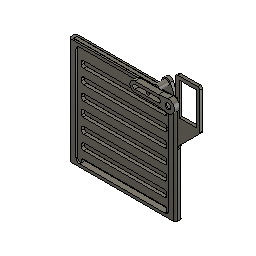
curtains (Autodesk Fusion 360 design; units mm, degrees)
Autodesk Fusion 360 part; units mm, degrees
note: some values were not read from the file. Chosen so that the rebuilt part matches the saved one: which bodies a step acts on; which face or edge a step refers to.
sketch "Sketch1" plane through (0, 0, 0) normal (0, 1, 0) x (1, 0, 0)
  line L0 (37.5, -2.5) -> (-37.5, -2.5)
  line L1 (-37.5, -2.5) -> (-37.5, 2.5)
  line L2 (-37.5, 2.5) -> (37.5, 2.5)
  line L3 (37.5, 2.5) -> (37.5, -2.5)
  line L4 (37.5, -2.5) -> (-37.5, 2.5) construction
  line L5 (-37.5, -2.5) -> (37.5, 2.5) construction
  dimension "d1" = 5
  dimension "d2" = 75
  constraint horizontal L0
  constraint perpendicular L0 L1
  constraint parallel L0 L2
  constraint parallel L1 L3
  constraint coincident L4 origin
  constraint coincident L5 origin
  measures "d1" distance of L0.end L1.end
  measures "d2" distance of L1.end L2.end
extrude "Extrude1" add sketch "Sketch1" along normal blind 75 makes body 1
sketch "Sketch2" plane through (0, 0, 2.5) normal (0, 0, 1) x (1, 0, 0)
  line L0 (-37.5, 0) -> (37.5, 0)
  line L1 (37.5, 0) -> (37.5, 75)
  line L2 (37.5, 75) -> (-37.5, 75)
  line L3 (-37.5, 75) -> (-37.5, 0)
  line L4 (-35.5, 2) -> (35.5, 2)
  line L5 (35.5, 2) -> (35.5, 73)
  line L6 (35.5, 73) -> (-35.5, 73)
  line L7 (-35.5, 73) -> (-35.5, 2)
  dimension "d5" = -2
extrude "Extrude2" cut sketch "Sketch2" against normal blind 3.8 contours L4 L5 L6 L7 bodies 1
sketch "Sketch3" plane through (0, 73, 0) normal (0, -1, 0) x (1, 0, 0)
  line L0 (35.5, 2.5) -> (-35.5, 2.5)
  line L1 (-35.5, 2.5) -> (-35.5, -1.3)
  line L2 (-35.5, -1.3) -> (35.5, -1.3)
  line L3 (35.5, -1.3) -> (35.5, 2.5)
  line L4 (35.5, 1.3) -> (-35.5, 1.3)
  dimension "d8" = 1.2
  constraint coincident L3 L4.start
  constraint coincident L1 L4.end
  constraint perpendicular L1 L4
  measures "d8" distance of L0 L4
extrude "Extrude3" cut sketch "Sketch3" against normal blind 5 contours L1 L2 L3 L4 bodies 1
sketch "Sketch4" plane through (0, 0, 2.5) normal (0, 0, 1) x (1, 0, 0)
  line L0 (35.5, 2) -> (-35.5, 2)
  line L1 (-35.5, 2) -> (-35.5, 73)
  line L2 (-35.5, 73) -> (35.5, 73)
  line L3 (35.5, 73) -> (35.5, 2)
  line L4 (-37.5, 0) -> (37.5, 0)
  line L5 (37.5, 0) -> (37.5, 75)
  line L6 (37.5, 75) -> (-37.5, 75)
  line L7 (-37.5, 75) -> (-37.5, 0)
  line L8 (-32.5, 73) -> (-32.5, 2)
  line L9 (32.5, 73) -> (32.5, 2)
  dimension "d11" = 3
  dimension "d12" = 3
  constraint coincident L2 L8.start
  constraint coincident L0 L8.end
  constraint perpendicular L0 L8
  constraint coincident L2 L9.start
  constraint coincident L0 L9.end
  constraint perpendicular L0 L9
  measures "d11" distance of L1 L8
  measures "d12" distance of L3 L9
extrude "Extrude4" add sketch "Sketch4" against normal blind 1.2 contours L0 L2 L3 L9 | L0 L1 L2 L8 bodies 1
sketch "Sketch5" plane through (0, 0, -1.3) normal (0, 0, 1) x (1, 0, 0)
  line L0 (-35.5, 75) -> (-35.5, 2)
  line L1 (-35.5, 2) -> (35.5, 2)
  line L2 (35.5, 2) -> (35.5, 75)
  line L3 (35.5, 75) -> (-35.5, 75)
  line L4 (-32.5, 73) -> (-32.5, 2)
  line L5 (32.5, 73) -> (32.5, 2)
  line L6 (32.5, 2) -> (-32.5, 2)
  line L7 (-32.5, 73) -> (32.5, 73)
  line L8 (0, 73) -> (0, 2) construction
  line L9 (30, 35) -> (-30, 35)
  line L10 (-30, 35) -> (-30, 40)
  line L11 (-30, 40) -> (30, 40)
  line L12 (30, 40) -> (30, 35)
  line L13 (30, 35) -> (-30, 40) construction
  line L14 (-30, 35) -> (30, 40) construction
  line L15 (30, 5) -> (-30, 5)
  line L16 (-30, 5) -> (-30, 10)
  line L17 (30, 10) -> (30, 5)
  line L18 (-30, 10) -> (30, 10)
  line L19 (30, 15) -> (-30, 15)
  line L20 (-30, 15) -> (-30, 20)
  line L21 (30, 20) -> (30, 15)
  line L22 (-30, 20) -> (30, 20)
  line L23 (30, 25) -> (-30, 25)
  line L24 (-30, 25) -> (-30, 30)
  line L25 (30, 30) -> (30, 25)
  line L26 (-30, 30) -> (30, 30)
  line L27 (30, 45) -> (-30, 45)
  line L28 (-30, 45) -> (-30, 50)
  line L29 (30, 50) -> (30, 45)
  line L30 (-30, 50) -> (30, 50)
  line L31 (30, 55) -> (-30, 55)
  line L32 (-30, 55) -> (-30, 60)
  line L33 (30, 60) -> (30, 55)
  line L34 (-30, 60) -> (30, 60)
  line L35 (30, 65) -> (-30, 65)
  line L36 (-30, 65) -> (-30, 70)
  line L37 (30, 70) -> (30, 65)
  line L38 (-30, 70) -> (30, 70)
  point P0 (0, 37.5)
  dimension "d15" = 60
  dimension "d16" = 5
  dimension "d19" = 0
  dimension "d20" = 10
  constraint midpoint L7 L8.start
  constraint midpoint L6 L8.end
  constraint horizontal L9
  constraint perpendicular L9 L10
  constraint parallel L9 L11
  constraint parallel L10 L12
  constraint coincident L13 P0
  constraint coincident L14 P0
  constraint midpoint L8 P0
  measures "d15" distance of L10.end L11.end
  measures "d16" distance of L9.end L10.end
extrude "Extrude5" cut sketch "Sketch5" against normal blind 5 contours L9 L10 L11 L12 | L15 L16 L17 L18 | L19 L20 L21 L22 | L23 L24 L25 L26 | L27 L28 L29 L30 | L31 L32 L33 L34 | L35 L36 L37 L38 bodies 1
fillet "Fillet1" radius 2.5 4 edges at (-32.5, 73, 1.9) (-32.5, 2, 1.9) (32.5, 73, 1.9) (32.5, 2, 1.9) on bodies 1
fillet "Fillet2" radius 1.5 4 edges at (-37.5, 37.5, 2.5) (-37.5, 37.5, -2.5) (37.5, 37.5, -2.5) (37.5, 37.5, 2.5) on bodies 1
fillet "Fillet3" radius 1.5 20 edges at (-30, 50, -1.9) (-30, 45, -1.9) (-30, 30, -1.9) (-30, 25, -1.9) (-30, 40, -1.9) (-30, 35, -1.9) (-30, 20, -1.9) (-30, 15, -1.9) (-30, 10, -1.9) (-30, 5, -1.9) (30, 50, -1.9) (30, 45, -1.9) (30, 30, -1.9) (30, 25, -1.9) (30, 40, -1.9) (30, 35, -1.9) (30, 20, -1.9) (30, 15, -1.9) (30, 10, -1.9) (30, 5, -1.9) on bodies 1
fillet "Fillet3" radius 1.5 8 edges at (-30, 55, -1.9) (-30, 60, -1.9) (-30, 65, -1.9) (-30, 70, -1.9) (30, 70, -1.9) (30, 65, -1.9) (30, 60, -1.9) (30, 55, -1.9) on bodies 1
sketch "Sketch6" plane through (0, 75, 0) normal (0, 1, 0) x (-1, 0, 0)
  arc A0 (-36, 2.5) -> (-37.5, 1) centre (-36, 1) ccw
  line L0 (-37.5, 1) -> (-37.5, -1)
  arc A1 (-37.5, -1) -> (-36, -2.5) centre (-36, -1) ccw
  line L1 (-36, -2.5) -> (36, -2.5)
  arc A2 (36, -2.5) -> (37.5, -1) centre (36, -1) ccw
  line L2 (37.5, -1) -> (37.5, 1)
  arc A3 (37.5, 1) -> (36, 2.5) centre (36, 1) ccw
  line L3 (36, 2.5) -> (-36, 2.5)
  line L4 (35.5, 1.3) -> (35.5, -1.3)
  line L5 (35.5, -1.3) -> (-35.5, -1.3)
  line L6 (-35.5, -1.3) -> (-35.5, 1.3)
  line L7 (-35.5, 1.3) -> (35.5, 1.3)
  line L8 (-35.3, 1.1) -> (35.3, 1.1)
  line L9 (35.3, 1.1) -> (35.3, -1.1)
  line L10 (35.3, -1.1) -> (-35.3, -1.1)
  line L11 (-35.3, -1.1) -> (-35.3, 1.1)
  dimension "d29" = 0.2
extrude "Extrude6" add sketch "Sketch6" against normal blind 73 separate body contours L8 L9 L10 L11 makes body 2
sketch "Sketch8" plane through (0, 0, 1.1) normal (0, 0, 1) x (1, 0, 0)
  line L0 (35.3, 75) -> (-35.3, 75)
  line L1 (-35.3, 75) -> (-35.3, 2)
  line L2 (-35.3, 2) -> (35.3, 2)
  line L3 (35.3, 2) -> (35.3, 75)
  line L4 (-28.5, 5) -> (28.5, 5)
  arc A0 (28.5, 5) -> (30, 6.5) centre (28.5, 6.5) ccw
  line L5 (30, 6.5) -> (30, 8.5)
  arc A1 (30, 8.5) -> (28.5, 10) centre (28.5, 8.5) ccw
  line L6 (28.5, 10) -> (-28.5, 10)
  arc A2 (-28.5, 10) -> (-30, 8.5) centre (-28.5, 8.5) ccw
  line L7 (-30, 8.5) -> (-30, 6.5)
  arc A3 (-30, 6.5) -> (-28.5, 5) centre (-28.5, 6.5) ccw
  line L8 (-28.5, 45) -> (28.5, 45)
  arc A4 (28.5, 45) -> (30, 46.5) centre (28.5, 46.5) ccw
  line L9 (30, 46.5) -> (30, 48.5)
  arc A5 (30, 48.5) -> (28.5, 50) centre (28.5, 48.5) ccw
  line L10 (28.5, 50) -> (-28.5, 50)
  arc A6 (-28.5, 50) -> (-30, 48.5) centre (-28.5, 48.5) ccw
  line L11 (-30, 48.5) -> (-30, 46.5)
  arc A7 (-30, 46.5) -> (-28.5, 45) centre (-28.5, 46.5) ccw
  line L12 (-28.5, 15) -> (28.5, 15)
  arc A8 (28.5, 15) -> (30, 16.5) centre (28.5, 16.5) ccw
  line L13 (30, 16.5) -> (30, 18.5)
  arc A9 (30, 18.5) -> (28.5, 20) centre (28.5, 18.5) ccw
  line L14 (28.5, 20) -> (-28.5, 20)
  arc A10 (-28.5, 20) -> (-30, 18.5) centre (-28.5, 18.5) ccw
  line L15 (-30, 18.5) -> (-30, 16.5)
  arc A11 (-30, 16.5) -> (-28.5, 15) centre (-28.5, 16.5) ccw
  line L16 (-28.5, 25) -> (28.5, 25)
  arc A12 (28.5, 25) -> (30, 26.5) centre (28.5, 26.5) ccw
  line L17 (30, 26.5) -> (30, 28.5)
  arc A13 (30, 28.5) -> (28.5, 30) centre (28.5, 28.5) ccw
  line L18 (28.5, 30) -> (-28.5, 30)
  arc A14 (-28.5, 30) -> (-30, 28.5) centre (-28.5, 28.5) ccw
  line L19 (-30, 28.5) -> (-30, 26.5)
  arc A15 (-30, 26.5) -> (-28.5, 25) centre (-28.5, 26.5) ccw
  line L20 (-30, 38.5) -> (-30, 36.5)
  arc A16 (-30, 36.5) -> (-28.5, 35) centre (-28.5, 36.5) ccw
  line L21 (-28.5, 35) -> (28.5, 35)
  arc A17 (28.5, 35) -> (30, 36.5) centre (28.5, 36.5) ccw
  line L22 (30, 36.5) -> (30, 38.5)
  arc A18 (30, 38.5) -> (28.5, 40) centre (28.5, 38.5) ccw
  line L23 (28.5, 40) -> (-28.5, 40)
  arc A19 (-28.5, 40) -> (-30, 38.5) centre (-28.5, 38.5) ccw
  line L24 (36, 75) -> (36, 0)
  line L25 (36, 0) -> (-36, 0)
  line L26 (-36, 0) -> (-36, 75)
  line L27 (-36, 75) -> (36, 75)
  line L28 (0, 45) -> (0, 30) construction
  line L29 (0, 25) -> (0, 40) construction
  line L30 (0, 35) -> (0, 20) construction
  line L31 (0, 15) -> (0, 10) construction
  line L32 (-30, 30.125) -> (30, 30.125)
  line L33 (30, 30.125) -> (30, 34.875)
  line L34 (30, 34.875) -> (-30, 34.875)
  line L35 (-30, 34.875) -> (-30, 30.125)
  line L36 (-30, 30.125) -> (30, 34.875) construction
  line L37 (30, 30.125) -> (-30, 34.875) construction
  line L38 (-30, 7.5) -> (30, 7.5) construction
  line L39 (30, 0.125) -> (30, 4.875)
  line L40 (30, 4.875) -> (-30, 4.875)
  line L41 (-30, 0.125) -> (30, 0.125)
  line L42 (-30, 4.875) -> (-30, 0.125)
  line L43 (30, 10.125) -> (30, 14.875)
  line L44 (30, 14.875) -> (-30, 14.875)
  line L45 (-30, 10.125) -> (30, 10.125)
  line L46 (-30, 14.875) -> (-30, 10.125)
  line L47 (30, 20.125) -> (30, 24.875)
  line L48 (30, 24.875) -> (-30, 24.875)
  line L49 (-30, 20.125) -> (30, 20.125)
  line L50 (-30, 24.875) -> (-30, 20.125)
  line L51 (30, 40.125) -> (30, 44.875)
  line L52 (30, 44.875) -> (-30, 44.875)
  line L53 (-30, 40.125) -> (30, 40.125)
  line L54 (-30, 44.875) -> (-30, 40.125)
  line L55 (30, 50.125) -> (30, 54.875)
  line L56 (30, 54.875) -> (-30, 54.875)
  line L57 (-30, 50.125) -> (30, 50.125)
  line L58 (-30, 54.875) -> (-30, 50.125)
  line L59 (30, 60.125) -> (30, 64.875)
  line L60 (30, 64.875) -> (-30, 64.875)
  line L61 (-30, 60.125) -> (30, 60.125)
  line L62 (-30, 64.875) -> (-30, 60.125)
  line L63 (30, 70.125) -> (30, 74.875)
  line L64 (30, 74.875) -> (-30, 74.875)
  line L65 (-30, 70.125) -> (30, 70.125)
  line L66 (-30, 74.875) -> (-30, 70.125)
  line L67 (-28.5, 65) -> (28.5, 65)
  line L68 (30, 66.5) -> (30, 68.5)
  line L69 (28.5, 70) -> (-28.5, 70)
  line L70 (-30, 68.5) -> (-30, 66.5)
  line L71 (-28.5, 55) -> (28.5, 55)
  line L72 (30, 56.5) -> (30, 58.5)
  line L73 (28.5, 60) -> (-28.5, 60)
  line L74 (-30, 58.5) -> (-30, 56.5)
  arc A20 (28.5, 65) -> (30, 66.5) centre (28.5, 66.5) ccw
  arc A21 (30, 68.5) -> (28.5, 70) centre (28.5, 68.5) ccw
  arc A22 (-28.5, 70) -> (-30, 68.5) centre (-28.5, 68.5) ccw
  arc A23 (-30, 66.5) -> (-28.5, 65) centre (-28.5, 66.5) ccw
  arc A24 (28.5, 55) -> (30, 56.5) centre (28.5, 56.5) ccw
  arc A25 (30, 58.5) -> (28.5, 60) centre (28.5, 58.5) ccw
  arc A26 (-28.5, 60) -> (-30, 58.5) centre (-28.5, 58.5) ccw
  arc A27 (-30, 56.5) -> (-28.5, 55) centre (-28.5, 56.5) ccw
  point P0 (0, 37.5)
  point P1 (0, 32.5)
  point P2 (0, 27.5)
  point P3 (0, 12.5)
  dimension "d36" = 4.75
  dimension "d39" = 60
  dimension "d54" = 0
  dimension "d55" = 10
  constraint midpoint L8 L28.start
  constraint midpoint L18 L28.end
  constraint midpoint L16 L29.start
  constraint midpoint L23 L29.end
  constraint midpoint L21 L30.start
  constraint midpoint L14 L30.end
  constraint midpoint L12 L31.start
  constraint midpoint L6 L31.end
  constraint midpoint L28 P0
  constraint horizontal L32
  constraint perpendicular L32 L33
  constraint parallel L32 L34
  constraint parallel L33 L35
  constraint coincident L36 P1
  constraint coincident L37 P1
  constraint midpoint L29 P1
  constraint midpoint L30 P2
  constraint midpoint L31 P3
  constraint midpoint L7 L38.start
  constraint midpoint L5 L38.end
  measures "d36" distance of L32.start L34.end
  measures "d39" distance of L33.end L34.end
extrude "Extrude8" cut sketch "Sketch8" against normal blind 2.2 contours L2 L39 L40 L42 | L32 L33 L34 L35 | L43 L44 L45 L46 | L47 L48 L49 L50 | L51 L52 L53 L54 | L55 L56 L57 L58 | L59 L60 L61 L62 bodies 2
fillet "Fillet4" radius 1 4 edges at (-30, 30.125, 0) (-30, 34.875, 0) (30, 34.875, 0) (30, 30.125, 0) on bodies 2
fillet "Fillet4" radius 1.5 22 edges at (-30, 24.875, 0) (-30, 20.125, 0) (-30, 14.875, 0) (-30, 10.125, 0) (-30, 4.875, 0) (30, 4.875, 0) (30, 10.125, 0) (30, 14.875, 0) (30, 20.125, 0) (30, 24.875, 0) (30, 44.875, 0) (30, 40.125, 0) (30, 54.875, 0) (30, 50.125, 0) (30, 64.875, 0) (30, 60.125, 0) (-30, 64.875, 0) (-30, 60.125, 0) (-30, 54.875, 0) (-30, 50.125, 0) (-30, 44.875, 0) (-30, 40.125, 0) on bodies 2
ref_plane "WorkPlane1" through (0, 37.5, 0) normal (0, 0, 1) x (1, 0, 0)
sketch "Sketch9" plane through (0, 25, 0) normal (0, 0, 1) x (1, 0, 0)
  line L0 (37.5, 50) -> (37.5, -25)
  line L1 (37.5, -25) -> (37.5, 50)
  line L2 (37.5, 50) -> (44.5, 50) construction
  line L3 (50.5, 38.5) -> (38.5, 38.5)
  line L4 (38.5, 38.5) -> (38.5, 61.5)
  line L5 (38.5, 61.5) -> (50.5, 61.5)
  line L6 (50.5, 61.5) -> (50.5, 38.5)
  line L7 (50.5, 38.5) -> (38.5, 61.5) construction
  line L8 (38.5, 38.5) -> (50.5, 61.5) construction
  line L9 (53, 36) -> (36, 36)
  line L10 (36, 36) -> (36, 64)
  line L11 (36, 64) -> (53, 64)
  line L12 (53, 64) -> (53, 36)
  point P0 (44.5, 50)
  dimension "d46" = 23
  dimension "d47" = 12
  dimension "d48" = 1
  dimension "d49" = -2.5
  constraint coincident L0.start L1.end
  constraint perpendicular L0 L2
  constraint horizontal L3
  constraint perpendicular L3 L4
  constraint parallel L3 L5
  constraint parallel L4 L6
  constraint coincident L7 P0
  constraint coincident L8 P0
  constraint coincident P0 L2.end
  measures "d46" distance of L3.start L5.end
  measures "d47" distance of L4.end L5.end
  measures "d48" distance of L1 L4
extrude "Extrude9" add sketch "Sketch9" along normal mid plane 2 bodies 1
chamfer "Chamfer1" distance 15.5 angle 45 1 edges at (37.5, 61, 0) on bodies 1
fillet "Fillet5" radius 5 1 edges at (37.5, 45.5031, 0) on bodies 1
fillet "Fillet6" radius 1.5 6 edges at (52.9984, 61, -1) (36, 89, 0) (52.9984, 61, 1) (52.9969, 61, 0) (53, 61, 0) (53, 89, 0) on bodies 1
sketch "Sketch10" plane through (0, 0, 1) normal (0, 0, 1) x (1, 0, 0)
  arc A0 (53, 87.5) -> (51.5, 89) centre (51.5, 87.5) ccw
  line L0 (51.5, 89) -> (37.5, 89)
  arc A1 (37.5, 89) -> (36, 87.5) centre (37.5, 87.5) ccw
  line L1 (36, 87.5) -> (36, 75)
  line L2 (36, 75) -> (37.5, 75)
  line L3 (37.5, 75) -> (37.5, 43.4289)
  arc A2 (38.9645, 46.9645) -> (37.5, 43.4289) centre (42.5, 43.4289) ccw
  line L4 (38.9645, 46.9645) -> (52.5607, 60.5607)
  line L5 (53, 61.6213) -> (53, 87.5)
  line L6 (38.5, 86.5) -> (50.5, 86.5)
  line L7 (50.5, 86.5) -> (50.5, 63.5)
  line L8 (50.5, 63.5) -> (38.5, 63.5)
  line L9 (38.5, 63.5) -> (38.5, 86.5)
  line L10 (44.5, 86.5) -> (44.5, 80.6)
  line L11 (44.5, 80.6) -> (29.5, 80.6) construction
  line L12 (35.3, 75) -> (-35.3, 75)
  line L13 (-35.3, 75) -> (35.3, 75)
  circle A3 centre (29.5, 80.6) radius 1
  circle A4 centre (29.5, 80.6) radius 3
  line L14 (35.3, 75) -> (32.2372, 81.8278)
  line L15 (29.5, 82.4332) -> (29.5, 78.4139) construction
  line L16 (23.7, 75) -> (26.7628, 81.8278)
  arc A5 (52.5607, 60.5607) -> (53, 61.6213) centre (51.5, 61.6213) ccw
  dimension "d65" = 15
  dimension "d66" = 5.9
  dimension "d67" = 2
  dimension "d68" = 2
  constraint midpoint L6 L10.start
  constraint perpendicular L6 L10
  constraint perpendicular L1 L11
  constraint coincident L11.end A3.centre
  constraint coincident L12.start L13.end
  constraint coincident A4 L14.end
  constraint tangent A4 L14
  constraint perpendicular L11 L15
  constraint symmetric L12.start L15 L16.start
  constraint symmetric L14.end L15 L16.end
  measures "d65" distance of L10.end L11.end
  measures "d66" distance of L6 L10.end
  measures "d67" diameter of A3
  measures "d68" distance of A3
extrude "Extrude10" add sketch "Sketch10" against normal blind 2.1 separate body contours L12 L13 A4 L14 L16 | A4 makes body 3
combine "Combine1" operation add target body 2 tool bodies 3
ref_plane "WorkPlane2" through (29.5, 79.3, 11) normal (0, 0, 1) x (1, 0, 0)
sketch "Sketch11" plane through (29.5, 79.3, 11) normal (0, 0, 1) x (1, 0, 0)
  circle A0 centre (0, 1.3) radius 1
  line L0 (9, 7.2) -> (21, 7.2)
  line L1 (9, -15.8) -> (9, 7.2)
  line L2 (21, -15.8) -> (9, -15.8)
  line L3 (21, 7.2) -> (21, -15.8)
  line L4 (15, 7.2) -> (15, 1.2) construction
  circle A1 centre (15, 1.2) radius 2.5
  line L5 (8.2797, 2.8) -> (-8.2797, 2.8)
  arc A2 (-8.2797, 2.8) -> (-8.2797, -0.2) centre (-8.2797, 1.3) ccw
  line L6 (-8.2797, -0.2) -> (8.2797, -0.2)
  arc A3 (8.2797, -0.2) -> (8.2797, 2.8) centre (8.2797, 1.3) ccw
  line L7 (8.2797, 1.3) -> (-8.2797, 1.3) construction
  line L8 (-8.2797, -2.2) -> (8.2797, -2.2)
  arc A4 (8.2797, -2.2) -> (8.2797, 4.8) centre (8.2797, 1.3) ccw
  line L9 (8.2797, 4.8) -> (-8.2797, 4.8)
  arc A5 (-8.2797, 4.8) -> (-8.2797, -2.2) centre (-8.2797, 1.3) ccw
  circle A6 centre (15, 1.2) radius 4.5
  line L10 (15, 5.7) -> (8.2797, 4.8)
  line L11 (15, -3.3) -> (8.2797, -2.2)
  point P0 (0, 1.3)
  dimension "d72" = 6
  dimension "d73" = 5
  dimension "d74" = 3
  dimension "d75" = 2
  dimension "d76" = 2
  constraint midpoint L0 L4.start
  constraint perpendicular L0 L4
  constraint coincident L4.end A1.centre
  constraint tangent L5 A2
  constraint tangent A2 L6
  constraint parallel L5 L6
  constraint tangent L6 A3
  constraint tangent L5 A3
  constraint horizontal L7
  constraint coincident P0 A0.centre
  constraint midpoint L7 P0
  constraint coincident A6 L10.start
  constraint coincident L4 L10.start
  constraint coincident A6 L11.start
  measures "d72" distance of L0 L4.end
  measures "d73" diameter of A1
  measures "d74" diameter of A2
extrude "Extrude11" add sketch "Sketch11" along normal blind 3 separate body contours L1 A4 A6 L10 | L1 A4 L10 | L1 A3 A4 A6 | L1 L5 A2 L6 A3 L8 A4 L9 A5 | A4 A6 L10 L11 | A4 A6 | L1 A4 L11 | L1 A4 A6 L11 makes body 4
sketch "Sketch12" plane through (0, 0, 14) normal (0, 0, 1) x (1, 0, 0)
  circle A0 centre (44.5, 80.5) radius 2.5
  arc A1 (37.7797, 79.1) -> (37.7797, 82.1) centre (37.7797, 80.6) ccw
  line L0 (37.7797, 79.1) -> (21.2203, 79.1)
  arc A2 (21.2203, 82.1) -> (21.2203, 79.1) centre (21.2203, 80.6) ccw
  line L1 (21.2203, 82.1) -> (37.7797, 82.1)
  line L2 (44.5, 85) -> (37.7797, 84.1)
  line L3 (37.7797, 84.1) -> (21.2203, 84.1)
  arc A3 (21.2203, 84.1) -> (21.2203, 77.1) centre (21.2203, 80.6) ccw
  line L4 (21.2203, 77.1) -> (37.7797, 77.1)
  line L5 (37.7797, 77.1) -> (44.5, 76)
  arc A4 (44.5, 76) -> (44.5, 85) centre (44.5, 80.5) ccw
  circle A5 centre (44.5, 80.5) radius 2
  dimension "d79" = 4
  constraint concentric A0 A5
  measures "d79" diameter of A5
extrude "Extrude12" add sketch "Sketch12" along normal blind 0.8 contours A0 | L2 L3 A3 L4 L5 A4 bodies 4
sketch "Sketch13" plane through (0, 0, 1) normal (0, 0, 1) x (1, 0, 0)
  circle A0 centre (29.5, 80.6) radius 1
  line L0 (35.3, 75) -> (32.2372, 81.8278)
  arc A1 (32.2372, 81.8278) -> (26.7628, 81.8278) centre (29.5, 80.6) ccw
  line L1 (26.7628, 81.8278) -> (23.7, 75)
  line L2 (23.7, 75) -> (35.3, 75)
  circle A2 centre (29.5, 80.6) radius 1
  circle A3 centre (29.5, 80.6) radius 2
  dimension "d82" = 2
  dimension "d83" = 4
  constraint concentric A0 A2
  constraint concentric A2 A3
  measures "d82" diameter of A2
  measures "d83" diameter of A3
extrude "Extrude13" add sketch "Sketch13" along normal blind 7 separate body contours A3 makes body 5
sketch "Sketch14" plane through (0, 0, 8) normal (0, 0, 1) x (1, 0, 0)
  circle A0 centre (29.5, 80.6) radius 1
  circle A1 centre (29.5, 80.6) radius 2
  circle A2 centre (29.5, 80.6) radius 1.25
  dimension "d86" = 2.5
  constraint concentric A0 A2
  measures "d86" diameter of A2
extrude "Extrude14" add sketch "Sketch14" along normal blind 6 contours A0 | A2 bodies 2 1 4 5
sketch "Sketch7" plane through (0, 0, -1.1) normal (0, 0, -1) x (-1, 0, 0)
  line L0 (22.8, 50) -> (-22.8, 50)
  line L1 (-22.8, 50) -> (-22.8, 2)
  line L2 (-22.8, 2) -> (22.8, 2)
  line L3 (22.8, 2) -> (22.8, 50)
  line L4 (17.5, 7) -> (-17.5, 7)
  arc A0 (-18.5, 8) -> (-17.5, 7) centre (-17.5, 8) ccw
  line L5 (-18.5, 8) -> (-18.5, 10)
  arc A1 (-17.5, 11) -> (-18.5, 10) centre (-17.5, 10) ccw
  line L6 (-17.5, 11) -> (17.5, 11)
  arc A2 (18.5, 10) -> (17.5, 11) centre (17.5, 10) ccw
  line L7 (18.5, 10) -> (18.5, 8)
  arc A3 (17.5, 7) -> (18.5, 8) centre (17.5, 8) ccw
  line L8 (17.5, 39) -> (-17.5, 39)
  arc A4 (-18.5, 40) -> (-17.5, 39) centre (-17.5, 40) ccw
  line L9 (-18.5, 40) -> (-18.5, 42)
  arc A5 (-17.5, 43) -> (-18.5, 42) centre (-17.5, 42) ccw
  line L10 (-17.5, 43) -> (17.5, 43)
  arc A6 (18.5, 42) -> (17.5, 43) centre (17.5, 42) ccw
  line L11 (18.5, 42) -> (18.5, 40)
  arc A7 (17.5, 39) -> (18.5, 40) centre (17.5, 40) ccw
  line L12 (17.5, 15) -> (-17.5, 15)
  arc A8 (-18.5, 16) -> (-17.5, 15) centre (-17.5, 16) ccw
  line L13 (-18.5, 16) -> (-18.5, 18)
  arc A9 (-17.5, 19) -> (-18.5, 18) centre (-17.5, 18) ccw
  line L14 (-17.5, 19) -> (17.5, 19)
  arc A10 (18.5, 18) -> (17.5, 19) centre (17.5, 18) ccw
  line L15 (18.5, 18) -> (18.5, 16)
  arc A11 (17.5, 15) -> (18.5, 16) centre (17.5, 16) ccw
  line L16 (17.5, 31) -> (-17.5, 31)
  arc A12 (-18.5, 32) -> (-17.5, 31) centre (-17.5, 32) ccw
  line L17 (-18.5, 32) -> (-18.5, 34)
  arc A13 (-17.5, 35) -> (-18.5, 34) centre (-17.5, 34) ccw
  line L18 (-17.5, 35) -> (17.5, 35)
  arc A14 (18.5, 34) -> (17.5, 35) centre (17.5, 34) ccw
  line L19 (18.5, 34) -> (18.5, 32)
  arc A15 (17.5, 31) -> (18.5, 32) centre (17.5, 32) ccw
  line L20 (18.5, 26) -> (18.5, 24)
  arc A16 (17.5, 23) -> (18.5, 24) centre (17.5, 24) ccw
  line L21 (17.5, 23) -> (-17.5, 23)
  arc A17 (-18.5, 24) -> (-17.5, 23) centre (-17.5, 24) ccw
  line L22 (-18.5, 24) -> (-18.5, 26)
  arc A18 (-17.5, 27) -> (-18.5, 26) centre (-17.5, 26) ccw
  line L23 (-17.5, 27) -> (17.5, 27)
  arc A19 (18.5, 26) -> (17.5, 27) centre (17.5, 26) ccw
  line L24 (-23.5, 50) -> (-23.5, 0)
  line L25 (-23.5, 0) -> (23.5, 0)
  line L26 (23.5, 0) -> (23.5, 50)
  line L27 (23.5, 50) -> (-23.5, 50)
extrude "Extrude7" [suppressed]
equation "d6 = -5.00 mm + 1.2 mm"
